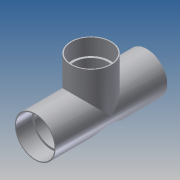
# Autodesk Inventor part: 2p5Tmod
Saved by Autodesk Inventor 2014 SP1 (Build 180222100, 222)
## iProperties
Company: HERA Project
Created: 2013-06-12
Part Number: 2p5Tmod
Material: PVC-Piping
Document SubType Name: Modeling
Designer: David DeBoer
Density: 1.4 g/cm^3
Description: modified 2" support pvc
Mass: 405.128 g
Surface Area: 960.349 cm^2
Volume: 289.377 cm^3
Appearance: Smooth - White
Author: David DeBoer
Title: sup
Autodesk Inventor part; units mm, degrees
ref_plane "YZ Plane" through (0, 0, 0) normal (1, 0, 0) x (0, 1, 0)
ref_plane "XZ Plane" through (0, 0, 0) normal (0, 1, 0) x (-1, 0, 0)
ref_plane "XY Plane" through (0, 0, 0) normal (0, 0, 1) x (1, 0, 0)
sketch "Sketch1" plane through (0, 0, 0) normal (0, 0, 1) x (1, 0, 0)
  circle A0 centre (0, 0) radius 31.75
  dimension "d0" = 63.5
  constraints: 1 centre point, 1 coincident
  measures "d0" diameter of A0
extrude "mainBody" add sketch "Sketch1" along normal blind 174.625
sketch "Sketch10" plane through (0, 0, 174.625) normal (0, 0, 1) x (1, 0, 0)
  circle A0 centre (0, 0) radius 30.1625 projected
  circle A1 centre (0, 0) radius 31.75 projected
  point P0 (0, 31.75)
  constraints: 1 vertical alignment, 1 other
ref_plane "Work Plane5" through (0, 31.75, 174.625) normal (0, 1, 0) x (-1, 0, 0)
sketch "Sketch11" plane through (0, 31.75, 174.625) normal (0, 1, 0) x (-1, 0, 0)
  circle A0 centre (0, -87.3125) radius 31.75
  line L0 (31.75, 0) -> (-31.75, 0) projected
  point P0 (0, -174.625)
  dimension "d29" = 87.3125
  dimension "d30" = 63.5
  constraints: 1 centre point
  measures "d29" distance from line of A0.centre L0
  measures "d30" diameter of A0
extrude "TBody" add sketch "Sketch11" along normal blind 38.1 and the other way blind 31.75
sketch "Sketch12" plane through (0, 69.85, 87.3125) normal (0, 1, 0) x (1, 0, 0)
  circle A0 centre (0, 0) radius 31.75 projected
  circle A1 centre (0, 0) radius 30.1625
  point P0 (0, 87.3125)
  dimension "d35" = 60.325
  constraints: 1 centre point, 1 coincident
  measures "d35" diameter of A1
extrude "TSocket" cut sketch "Sketch12" against normal blind 25.4 contours A1
sketch "Sketch13" plane through (0, 44.45, 87.3125) normal (0, 1, 0) x (1, 0, 0)
  circle A0 centre (0, 0) radius 30.1625 projected
  circle A1 centre (0, 0) radius 26.67
  point P0 (0, 87.3125)
  dimension "d39" = 53.34
  constraints: 1 centre point, 1 coincident
  measures "d39" diameter of A1
extrude "TTube" cut sketch "Sketch13" against normal blind 38.1 contours A1
sketch "Sketch14" plane through (0, 0, 174.625) normal (0, 0, 1) x (1, 0, 0)
  circle A0 centre (0, 0) radius 31.75 projected
  circle A1 centre (0, 0) radius 26.67
  dimension "d43" = 53.34
  constraints: 1 centre point, 1 coincident
  measures "d43" diameter of A1
extrude "mainTube" cut sketch "Sketch14" against normal blind 177.8 contours A1
sketch "Sketch15" plane through (0, 0, 174.625) normal (0, 0, 1) x (1, 0, 0)
  circle A0 centre (0, 0) radius 26.67 projected
  circle A1 centre (0, 0) radius 31.75 projected
  circle A2 centre (0, 0) radius 30.1625
  dimension "d47" = 60.325
  constraints: 1 centre point, 1 coincident
  measures "d47" diameter of A2
extrude "mainSocket1" cut sketch "Sketch15" against normal blind 25.4 contours A2
sketch "Sketch16" plane through (0, 0, 0) normal (0, 0, -1) x (-1, 0, 0)
  circle A0 centre (0, 0) radius 26.67 projected
  circle A1 centre (0, 0) radius 31.75 projected
  circle A2 centre (0, 0) radius 30.1625
  dimension "d51" = 60.325
  constraints: 1 centre point, 1 coincident
  measures "d51" diameter of A2
extrude "mainSocket2" cut sketch "Sketch16" against normal blind 25.4 contours A2
sketch "Sketch23" plane through (0, 0, 174.625) normal (0, 0, 1) x (1, 0, 0)
  circle A0 centre (0, 0) radius 30.1625 projected
  circle A1 centre (0, 0) radius 31.75 projected
  line L0 (0, 0) -> (-47.7364, 17.3746)
  line L1 (0, 0) -> (50.8, 0) construction
  line L2 (-58.8754, -11.0073) -> (-5.3744, -30.48)
  line L3 (-5.3744, -30.48) -> (50.8, -30.48)
  line L4 (-26.122, 21.0613) -> (-40.26, -17.7827)
  point P0 (-29.8352, 10.8591)
  dimension "d67" = 50.8
  dimension "d68" = 160
  dimension "d69" = 30.48
  constraints: 10 end point, 3 point on line, 1 equal length, 1 horizontal, 1 perpendicular, 1 tangent, 1 other
  measures "d67" distance of L0.start L0.end
  measures "d68" angle of L1 L0
  measures "d69" distance between parallel lines of L2 L0
ref_plane "Work Plane9" through (-29.8352, 10.8591, 174.625) normal (-0.9396926, 0.3420201, 0) x (-0.3420201, -0.9396926, 0)
sketch "Sketch24" plane through (-29.8352, 10.8591, 174.625) normal (-0.9396926, 0.3420201, 0) x (-0.3420201, -0.9396926, 0)
  circle A0 centre (31.75, -87.3125) radius 30.48
  point P0 (0, -174.625)
  dimension "d70" = 60.96
  constraints: 1 centre point
  measures "d70" diameter of A0
extrude "Extrusion18" cut sketch "Sketch24" along normal mid plane 203.2
sketch "Sketch25" plane through (0, 69.85, 87.3125) normal (0, 1, 0) x (1, 0, 0)
  circle A0 centre (0, 0) radius 31.75 projected
  circle A1 centre (-33.3789, 0) radius 1.6289
  point P0 (0, 87.3125)
  constraints: 1 centre point, 1 tangent
extrude "Extrusion19" add sketch "Sketch25" against normal blind 101.6 contours A1
sketch "Sketch26" plane through (-33.3789, 69.85, 87.3125) normal (0, 1, 0) x (1, 0, 0)
  circle A0 centre (0, 0) radius 1.6289 projected
  point P0 (1.6289, 0)
  point P1 (33.3789, 87.3125)
  constraints: 1 horizontal alignment
extrude "Extrusion20" cut sketch "Sketch26" against normal blind 12.7
body "Solid1"
